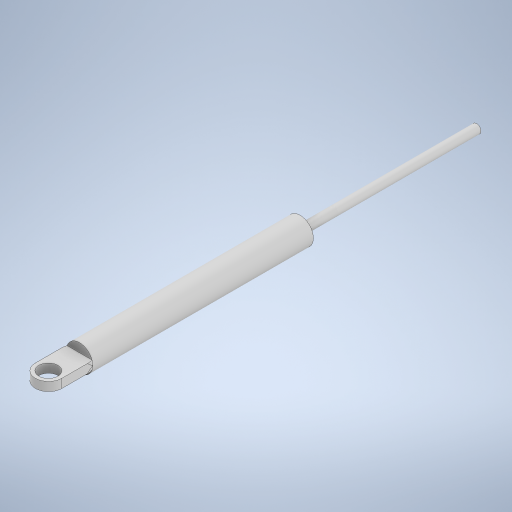
# Autodesk Inventor part: üst şaft part1
Saved by Autodesk Inventor 2023 (Build 270158000, 158)
## iProperties
Created: 2023-02-07
Part Number: üst şaft part1
Material: Generic
Document SubType Name: Modeling
Designer: omuru
Density: 1 g/cm^3
Appearance: Default
Author: omuru
Autodesk Inventor part; units mm, degrees
ref_plane "YZ Plane" through (0, 0, 0) normal (1, 0, 0) x (0, 1, 0)
ref_plane "XZ Plane" through (0, 0, 0) normal (0, 1, 0) x (-1, 0, 0)
ref_plane "XY Plane" through (0, 0, 0) normal (0, 0, 1) x (1, 0, 0)
sketch "Sketch1" plane through (0, 0, 0) normal (0, 0, 1) x (1, 0, 0)
  circle A0 centre (0, 0) radius 1.5
  dimension "d0" = 3
  constraints: 1 centre point, 1 coincident
  measures "d0" diameter of A0
extrude "Extrusion1" add sketch "Sketch1" against normal blind 25
sketch "Sketch2" plane through (0, 0, 0) normal (0, 1, 0) x (-1, 0, 0)
  line L0 (1.5, 0) -> (1.5, -25) projected
  line L1 (1.5, 0) -> (-1.5, 0)
  line L2 (-1.5, 0) -> (-1.5, -25) projected
  line L3 (0, 0) -> (0, 3.53)
  circle A0 centre (0, 3.53) radius 1.075
  line L4 (1.5, 0) -> (-1.5, 0)
  line L5 (-1.5, 0) -> (-1.5, 5)
  line L6 (-1.5, 5) -> (1.5, 5)
  line L7 (1.5, 5) -> (1.5, 0)
  dimension "d3" = 3.53
  dimension "d4" = 2.15
  dimension "d5" = 3
  dimension "d6" = 5
  constraints: 12 end point, 2 horizontal, 2 parallel, 2 point on line, 1 centre point, 1 coincident, 1 perpendicular, 1 vertical
  measures "d3" distance of L3.start L3.end
  measures "d4" diameter of A0
  measures "d5" distance of L5.end L6.end
  measures "d6" distance of L4.end L5.end
extrude "Extrusion2" add sketch "Sketch2" along normal mid plane 1
fillet "Fillet1" radius 1.5 2 edges at (1.5, 0, 5) (-1.5, 0, 5)
fillet "Fillet2" radius 1 4 edges at (1.5, 0.25, 0) (1.5, -0.25, 0) (-1.5, 0.25, 0) (-1.5, -0.25, 0)
sketch "Sketch3" plane through (0, 0, -25) normal (0, 0, -1) x (-1, 0, 0)
  circle A0 centre (0, 0) radius 0.5
  dimension "d11" = 1
  constraints: 1 centre point, 1 coincident
  measures "d11" diameter of A0
extrude "Extrusion3" add sketch "Sketch3" along normal blind 20
body "Solid1"
